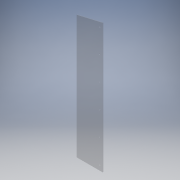
# Autodesk Inventor part: Side Walls
Saved by Autodesk Inventor 2017 (Build 210142000, 142)
## iProperties
Created: 2017-01-16
Part Number: Side Walls
Material: Polycarbonate, Clear
Document SubType Name: Modeling
Designer: Ben
Density: 1.2 g/cm^3
Appearance: Polycarbonate - Clear
Mass: 65.9067 g
Surface Area: 707.861 cm^2
Volume: 54.9223 cm^3
Author: Ben
Autodesk Inventor part; units mm, degrees
ref_plane "YZ Plane" through (0, 0, 0) normal (1, 0, 0) x (0, 1, 0)
ref_plane "XZ Plane" through (0, 0, 0) normal (0, 1, 0) x (-1, 0, 0)
ref_plane "XY Plane" through (0, 0, 0) normal (0, 0, 1) x (1, 0, 0)
sketch "Sketch1" plane through (0, 0, 0) normal (0, 0, 1) x (1, 0, 0)
  line L0 (0, 0) -> (82.55, 0)
  line L1 (82.55, 0) -> (82.55, 412.75)
  line L2 (82.55, 412.75) -> (0, 412.75)
  line L3 (0, 412.75) -> (0, 0)
  line L4 (73.025, 412.75) -> (73.025, 0) construction
  circle A0 centre (73.025, 15.875) radius 1.5875
  circle A1 centre (73.025, 92.075) radius 1.5875
  circle A2 centre (73.025, 168.275) radius 1.5875
  circle A3 centre (73.025, 244.475) radius 1.5875
  circle A4 centre (73.025, 320.675) radius 1.5875
  circle A5 centre (73.025, 396.875) radius 1.5875
  line L5 (82.55, 206.375) -> (0, 206.375) construction
  dimension "d0" = 82.55
  dimension "d1" = 412.75
  dimension "d7" = 9.525
  dimension "d8" = 3.175
  dimension "d11" = 76.2
  constraints: 12 end point, 6 centre point, 3 point on line, 2 midpoint, 2 parallel, 2 perpendicular, 1 horizontal, 1 vertical, 11 other
  measures "d0" distance of L0.start L0.end
  measures "d1" distance of L2.end L0.start
  measures "d7" distance of L0.end L4.end
  measures "d8" diameter of A0
  measures "d11" distance of A0.centre A1.centre
extrude "Extrusion1" add sketch "Sketch1" along normal blind 1.5875
chamfer "Chamfer1" distance 82.55 angle 13 1 edges at (0, 412.75, 0.7937) measured on face at (0.5, 412.75, 0.7938)
body "Solid1"
